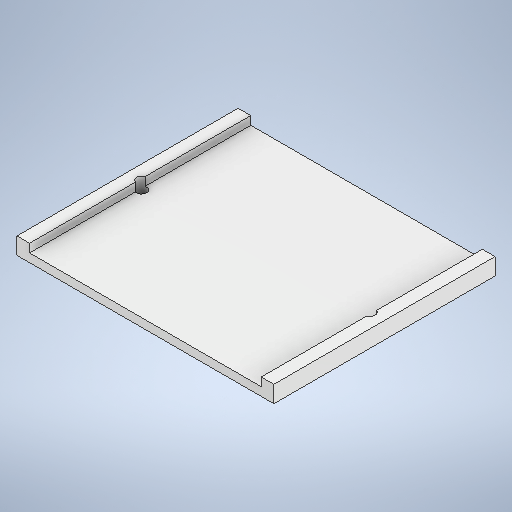
# Autodesk Inventor part: Module Holder Full Cover V1
Saved by Autodesk Inventor 2025 (Build 290162000, 162)
## iProperties
Created: 2024-03-20
Part Number: Module Holder Full Cover V1
Material: ABS Plastic
Document SubType Name: Modeling
Designer: cfang
Density: 1.06 g/cm^3
Appearance: Smooth - White
Author: cfang
Autodesk Inventor part; units mm, degrees
ref_plane "YZ Plane" through (0, 0, 0) normal (1, 0, 0) x (0, 1, 0)
ref_plane "XZ Plane" through (0, 0, 0) normal (0, 1, 0) x (-1, 0, 0)
ref_plane "XY Plane" through (0, 0, 0) normal (0, 0, 1) x (1, 0, 0)
sketch "Sketch1" plane through (0, 0, 0) normal (0, 1, 0) x (-1, 0, 0)
  line L0 (-30.5, -26.25) -> (30.5, -26.25)
  line L1 (30.5, -26.25) -> (30.5, 26.25)
  line L2 (30.5, 26.25) -> (-30.5, 26.25)
  line L3 (-30.5, 26.25) -> (-30.5, -26.25)
  line L4 (-30.5, -26.25) -> (30.5, 26.25) construction
  line L5 (30.5, -26.25) -> (-30.5, 26.25) construction
  point P0 (0, 0)
  dimension "d0" = 52.5
  dimension "d1" = 61
  constraints: 12 end point, 2 midpoint, 2 parallel, 1 horizontal, 1 perpendicular
  measures "d0" distance of L0.end L1.end
  measures "d1" distance of L1.end L2.end
extrude "Extrusion1" add sketch "Sketch1" along normal blind 4
sketch "Sketch2" plane through (0, 4, 0) normal (0, 1, 0) x (1, 0, 0)
  line L0 (-30.5, -26.25) -> (30.5, -26.25) projected
  line L1 (27.5, 26.25) -> (-30.5, 26.25)
  line L2 (-30.5, 26.25) -> (-30.5, -26.25)
  line L3 (-30.5, -26.25) -> (27.5, -26.25)
  line L4 (27.5, -26.25) -> (27.5, 26.25)
  line L5 (-30.5, 26.25) -> (-30.5, -26.25) projected
  line L6 (30.5, -26.25) -> (30.5, 26.25) projected
  line L7 (30.5, 26.25) -> (-30.5, 26.25) projected
  line L8 (-27.5, 26.25) -> (-27.5, -26.25)
  point P0 (0, 0)
  point P1 (27.5, -26.25)
  point P2 (-30.5, 0)
  point P3 (-27.5, -26.25)
  dimension "d26" = 3
  dimension "d29" = 3
  constraints: 10 end point, 5 point on line, 2 parallel, 2 perpendicular, 1 horizontal, 1 midpoint
  measures "d26" distance between parallel lines of L6 L4
  measures "d29" distance between parallel lines of L8 L2
extrude "Extrusion2" cut sketch "Sketch2" against normal blind 2 contours L8 L1 L4 L0
sketch "Sketch4" plane through (0, 0, 0) normal (0, -1, 0) x (1, 0, 0)
  line L0 (30.5, 26.25) -> (30.5, -26.25) projected
  line L1 (-30.5, -26.25) -> (-30.5, 26.25) projected
  point P0 (0, 0)
  point P1 (27.15, 0)
  point P2 (-27.15, 0)
  dimension "d28" = 3.35
  dimension "d30" = 3.35
  constraints: 1 horizontal alignment
  measures "d28" distance from line of point (27.15, 0) L0
  measures "d30" distance from line of L1 point (-27.15, 0)
hole "Hole2" at (27.15, 0, 0) at (-27.15, 0, 0) direction (0, 1, 0) diameter 2.4 end through all countersink diameter 3 countersink angle 90 clearance for "Flat Head Machine Screw" size "M2" standard "Ansi Metric M Profile"
equation "\"d29\" = d26"
equation "\"d30\" = d28"
body "Solid1"
